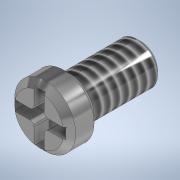
# Autodesk Inventor part: Parafuso 2,031
Saved by Autodesk Inventor 2021 (Build 250183000, 183)
## iProperties
Created: 2020-12-05
Part Number: Parafuso 2,031
Material: Liga de Nickel-Copper 400
Document SubType Name: Modeling
Designer: Bruno
Density: 8.83 g/cm^3
Appearance: Cromado - Preto polido
Author: Bruno
Autodesk Inventor part; units mm, degrees
ref_plane "YZ Plane" through (0, 0, 0) normal (1, 0, 0) x (0, 1, 0)
ref_plane "XZ Plane" through (0, 0, 0) normal (0, 1, 0) x (-1, 0, 0)
ref_plane "XY Plane" through (0, 0, 0) normal (0, 0, 1) x (1, 0, 0)
sketch "Esboço1" plane through (0, 0, 0) normal (0, 0, 1) x (1, 0, 0)
  circle A0 centre (0, 0) radius 1.0155
  dimension "d0" = 2.031
  constraints: 1 centre point, 1 coincident
  measures "d0" diameter of A0
extrude "Extrusão1" add sketch "Esboço1" against normal blind 3.5
sketch "Esboço2" plane through (0, 0, 0) normal (0, 0, 1) x (1, 0, 0)
  circle A0 centre (0, 0) radius 1.5
  dimension "d3" = 3
  constraints: 1 centre point, 1 coincident
  measures "d3" diameter of A0
extrude "Extrusão2" add sketch "Esboço2" along normal blind 1.5
sketch "Esboço3" plane through (0, 0, 1.5) normal (0, 0, 1) x (1, 0, 0)
  line L0 (-0.25, -1.25) -> (0.25, -1.25)
  line L1 (0.25, -1.25) -> (0.25, 1.25)
  line L2 (0.25, 1.25) -> (-0.25, 1.25)
  line L3 (-0.25, 1.25) -> (-0.25, -1.25)
  line L4 (-0.25, -1.25) -> (0.25, 1.25) construction
  line L5 (0.25, -1.25) -> (-0.25, 1.25) construction
  line L6 (-1.25, -0.25) -> (1.25, -0.25)
  line L7 (1.25, -0.25) -> (1.25, 0.25)
  line L8 (1.25, 0.25) -> (-1.25, 0.25)
  line L9 (-1.25, 0.25) -> (-1.25, -0.25)
  line L10 (-1.25, -0.25) -> (1.25, 0.25) construction
  line L11 (1.25, -0.25) -> (-1.25, 0.25) construction
  point P0 (0, 0)
  point P1 (-0.25, 0.25)
  point P2 (-0.25, -0.25)
  point P3 (0.25, -0.25)
  point P4 (0.25, 0.25)
  dimension "d6" = 0.5
  dimension "d7" = 2.5
  dimension "d8" = 2.5
  dimension "d9" = 0.5
  constraints: 24 end point, 4 midpoint, 4 parallel, 2 horizontal, 2 perpendicular
  measures "d6" distance between parallel lines of L3 L1
  measures "d7" distance between parallel lines of L0 L2
  measures "d8" distance between parallel lines of L9 L7
  measures "d9" distance between parallel lines of L6 L8
extrude "Extrusão3" cut sketch "Esboço3" against normal blind 0.75
thread "Rosca1" size "M2.2x0.45" class "6g" standard "ANSI Metric M Profile" full length
fillet "Arredondamento3" radius 0.2 4 edges at (-0.25, 0.25, 1.125) (0.25, 0.25, 1.125) (-0.25, -0.25, 1.125) (0.25, -0.25, 1.125)
chamfer "Chanfro1" distance 0.3 angle 45 2 edges at (-1.5, 0, 1.5) (-1.5, 0, 0)
chamfer "Chanfro2" distance 0.2 angle 45 1 edges at (-1.0155, 0, -3.5)
